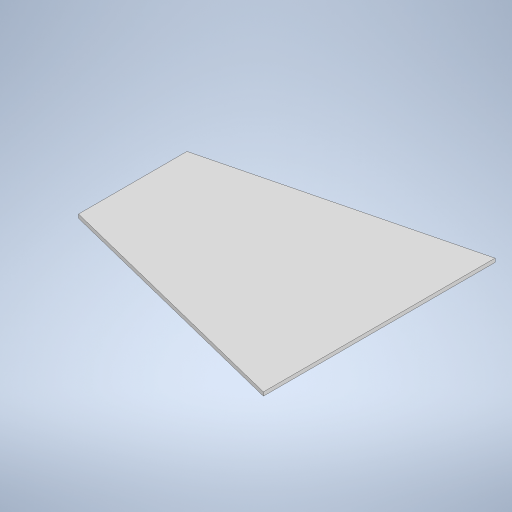
# Autodesk Inventor part: AI-TopPlateRS3
Saved by Autodesk Inventor 2024.3 (Build 283343000, 343)
## iProperties
Created: 2025-06-13
Part Number: AI-TopPlateRS3
Material: Generic
Document SubType Name: Modeling
Designer: ajclo
Density: 1 g/cm^3
Appearance: Default
Author: ajclo
Autodesk Inventor part; units mm, degrees
ref_plane "YZ Plane" through (0, 0, 0) normal (1, 0, 0) x (0, 1, 0)
ref_plane "XZ Plane" through (0, 0, 0) normal (0, 1, 0) x (-1, 0, 0)
ref_plane "XY Plane" through (0, 0, 0) normal (0, 0, 1) x (1, 0, 0)
sketch "Sketch1" plane through (0, 0, 0) normal (0, 1, 0) x (-1, 0, 0)
  line L0 (100, 94) -> (-100, 94)
  line L1 (-100, 94) -> (-100, -94)
  line L2 (-100, -94) -> (100, -94)
  line L3 (100, -94) -> (100, 94)
  line L4 (100, 94) -> (-100, -94) construction
  line L5 (-100, 94) -> (100, -94) construction
  line L6 (-100, 94) -> (100, 44)
  line L7 (100, -44) -> (-100, -94)
  point P0 (0, 0)
  point P1 (-100, -94)
  dimension "d0" = 188
  dimension "d1" = 200
  dimension "d2" = 50
  dimension "d3" = 50
  dimension "d4" = 0
  constraints: 16 end point, 2 midpoint, 2 parallel, 2 point on line, 1 horizontal, 1 perpendicular
  measures "d0" distance of L2.end L0.start
  measures "d1" distance of L1.end L2.end
  measures "d2" distance from line of L0 L6.end
  measures "d3" distance from line of L2 L7.start
  measures "d4" distance of L1.end L7.end
extrude "Extrusion1" add sketch "Sketch1" along normal blind 3 contours L6 L3 L7 L1
body "Solid1"
